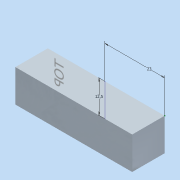
# Autodesk Inventor part: Cuvette
Saved by Autodesk Inventor 2015 (Build 190159000, 159)
## iProperties
Created: 2014-12-28
Part Number: Cuvette
Material: Glass
Document SubType Name: Modeling
Designer: Openlab
Density: 2.18 g/cm^3
Appearance: Clear
Author: Openlab
Autodesk Inventor part; units mm, degrees
ref_plane "YZ Plane" through (0, 0, 0) normal (1, 0, 0) x (0, 1, 0)
ref_plane "XZ Plane" through (0, 0, 0) normal (0, 1, 0) x (-1, 0, 0)
ref_plane "XY Plane" through (0, 0, 0) normal (0, 0, 1) x (1, 0, 0)
sketch "Sketch1" plane through (0, 0, 0) normal (0, 1, 0) x (-1, 0, 0)
  line L0 (45, 0) -> (0, 0)
  line L1 (0, 0) -> (0, -12.5)
  line L2 (0, -12.5) -> (45, -12.5)
  line L3 (45, -12.5) -> (45, 0)
  dimension "d0" = 45
  dimension "d1" = 12.5
  constraints: 8 end point, 2 parallel, 1 coincident, 1 horizontal, 1 perpendicular
  measures "d0" distance of L2.end L1.end
  measures "d1" distance of L1.end L0.end
extrude "Extrusion1" add sketch "Sketch1" along normal blind 12.5
sketch "Sketch2" plane through (0, 12.5, 0) normal (0, 1, 0) x (1, 0, 0)
  line L0 (-23, 0) -> (-23, 12.5)
  line L1 (-42.4869, 1.9235) -> (-42.4869, 10.7955) construction
  line L2 (-42.4869, 10.7955) -> (-38.8394, 10.7955) construction
  line L3 (-38.8394, 10.7955) -> (-38.8394, 1.9235) construction
  line L4 (-38.8394, 1.9235) -> (-42.4869, 1.9235) construction
  point P0 (0, 0)
  dimension "d4" = 12.5
  dimension "d5" = 23
  constraints: 2 end point, 1 vertical, 2 other
  measures "d4" distance of L0.start L0.end
  measures "d5" distance from line of point (0, 0) L0
body "Solid1"
